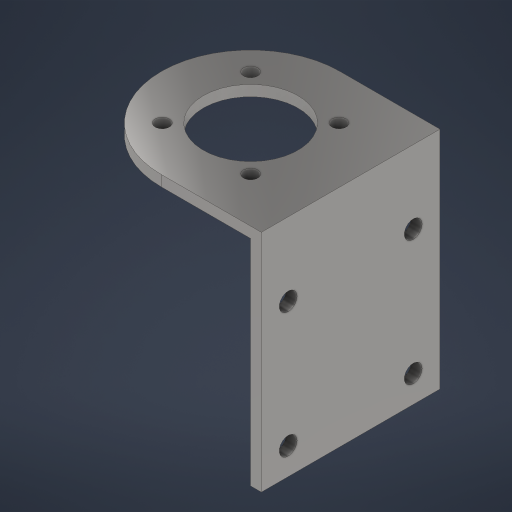
# Autodesk Inventor part: Foundation-Motor-Mount
Saved by Autodesk Inventor 2023 (Build 270158000, 158)
## iProperties
Created: 2023-09-15
Part Number: Foundation-Motor-Mount
Material: Steel, Mild
Document SubType Name: Modeling
Designer: Abhinav
Density: 7.85 g/cm^3
Appearance: Semi-Polished
Author: Abhinav
Autodesk Inventor part; units mm, degrees
ref_plane "YZ Plane" through (0, 0, 0) normal (1, 0, 0) x (0, 1, 0)
ref_plane "XZ Plane" through (0, 0, 0) normal (0, 1, 0) x (-1, 0, 0)
ref_plane "XY Plane" through (0, 0, 0) normal (0, 0, 1) x (1, 0, 0)
sketch "Sketch1" plane through (0, 0, 0) normal (0, 1, 0) x (-1, 0, 0)
  circle A0 centre (0, 0) radius 13.25
  line L0 (0, 0) -> (12.3744, 12.3744) construction
  line L1 (0, 0) -> (17.5, 0) construction
  line L2 (0, 0) -> (-12.3744, -12.3744) construction
  line L3 (0, 0) -> (17.5, 0) construction
  circle A1 centre (-12.3744, -12.3744) radius 2
  circle A2 centre (12.3744, 12.3744) radius 2
  circle A3 centre (12.3744, -12.3744) radius 2
  circle A4 centre (-12.3744, 12.3744) radius 2
  circle A5 centre (0, 0) radius 17.5 construction
  arc A6 (0, -25) -> (0, 25) centre (0, 0) ccw
  line L4 (0, 25) -> (-25, 25)
  line L5 (-25, 25) -> (-25, -25)
  line L6 (-25, -25) -> (0, -25)
  line L7 (-25, 25) -> (-28, 25)
  line L8 (-28, 25) -> (-28, -25)
  line L9 (-28, -25) -> (-25, -25)
  line L10 (-25, -25) -> (-25, 25)
  dimension "d0" = 26.5
  dimension "d1" = 17.5
  dimension "d2" = 45
  dimension "d3" = 17.5
  dimension "d4" = 135
  dimension "d5" = 4
  dimension "d6" = 4
  dimension "d7" = 50
  dimension "d10" = 3
  constraints: 22 end point, 6 centre point, 5 coincident, 4 horizontal, 3 parallel, 2 equal length, 2 perpendicular, 2 point on circle, 2 symmetric about line, 6 other
  measures "d0" diameter of A0
  measures "d1" distance of L1.start L0.end
  measures "d2" angle of L1 L0
  measures "d3" distance of L1.start L2.end
  measures "d4" angle of L2 L3
  measures "d5" diameter of A1
  measures "d6" diameter of A2
  measures "d7" diameter of A6
  measures "d10" distance of L9.end L8.end
extrude "Extrusion1" add sketch "Sketch1" along normal blind 3 contours L6 L5 L4 A6
extrude "Extrusion2" add sketch "Sketch1" along normal blind 3 and the other way blind 60 contours L9 L8 L7 L5
sketch "Sketch2" plane through (25, 0, -25) normal (-1, 0, 0) x (0, 0, 1)
  line L0 (50, -60) -> (50, 0) construction
  line L1 (0, -10) -> (50, -60) construction
  line L2 (7.5, -17.5) -> (42.5, -17.5) construction
  line L3 (42.5, -17.5) -> (42.5, -52.5) construction
  line L4 (42.5, -52.5) -> (7.5, -52.5) construction
  line L5 (7.5, -52.5) -> (7.5, -17.5) construction
  line L6 (7.5, -17.5) -> (42.5, -52.5) construction
  line L7 (42.5, -17.5) -> (7.5, -52.5) construction
  circle A0 centre (7.5, -17.5) radius 2.5
  circle A1 centre (42.5, -17.5) radius 2.5
  circle A2 centre (42.5, -52.5) radius 2.5
  circle A3 centre (7.5, -52.5) radius 2.5
  point P0 (25, 0)
  point P1 (25, -35)
  dimension "d15" = 35
  dimension "d16" = 35
  dimension "d17" = 5
  constraints: 14 end point, 4 centre point, 4 coincident, 3 equal radius, 3 midpoint, 2 parallel, 1 horizontal, 1 perpendicular
  measures "d15" distance of L3.end L4.end
  measures "d16" distance of L2.end L3.end
  measures "d17" diameter of A0
extrude "Extrusion3" cut sketch "Sketch2" against normal blind 5
body "Solid1"
